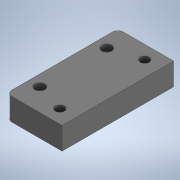
# Autodesk Inventor part: Stationaryjaw
Saved by Autodesk Inventor 2020.2 (Build 242310000, 310)
## iProperties
Created: 2021-06-22
Part Number: Stationaryjaw
Material: Generic
Document SubType Name: Modeling
Designer: JK
Density: 1 g/cm^3
Appearance: Gray
Author: JK
Autodesk Inventor part; units mm, degrees
ref_plane "YZ Plane" through (0, 0, 0) normal (1, 0, 0) x (0, 1, 0)
ref_plane "XZ Plane" through (0, 0, 0) normal (0, 1, 0) x (-1, 0, 0)
ref_plane "XY Plane" through (0, 0, 0) normal (0, 0, 1) x (1, 0, 0)
sketch "Sketch1" plane through (0, 0, 0) normal (0, 1, 0) x (-1, 0, 0)
  line L0 (25, 50) -> (-25, 50)
  line L1 (-25, 50) -> (-25, -50)
  line L2 (-25, -50) -> (25, -50)
  line L3 (25, -50) -> (25, 50)
  line L4 (25, 50) -> (-25, -50) construction
  line L5 (-25, 50) -> (25, -50) construction
  circle A0 centre (-11, 38) radius 6.5
  circle A1 centre (-11, -38) radius 6.5
  point P0 (0, 0)
  dimension "d0" = 13
  dimension "d1" = 100
  dimension "d2" = 50
  dimension "d3" = 14
  dimension "d4" = 12
  dimension "d5" = 12
  constraints: 12 end point, 2 centre point, 2 midpoint, 2 parallel, 1 equal radius, 1 horizontal, 1 perpendicular, 1 vertical alignment
  measures "d0" diameter of A0
  measures "d1" distance of L2.end L0.start
  measures "d2" distance of L1.end L2.end
  measures "d3" distance from line of A0.centre L1
  measures "d4" distance from line of L0 A0.centre
  measures "d5" distance from line of L2 A1.centre
extrude "Extrusion1" add sketch "Sketch1" along normal blind 20
sketch "Sketch2" plane through (0, 20, 0) normal (0, 1, 0) x (1, 0, 0)
  circle A0 centre (11, -38) radius 6.5 projected
  circle A1 centre (11, -38) radius 4
  circle A2 centre (11, 38) radius 6.5 projected
  circle A3 centre (11, 38) radius 4
  point P0 (0, 0)
  dimension "d8" = 8
  dimension "d9" = 8
  constraints: 2 centre point, 2 coincident
  measures "d8" diameter of A1
  measures "d9" diameter of A3
extrude "Extrusion2" add sketch "Sketch2" against normal blind 5
sketch "Sketch3" plane through (0, 0, 0) normal (0, -1, 0) x (1, 0, 0)
  circle A0 centre (-15, -30) radius 2.65
  circle A1 centre (-15, 30) radius 2.65
  line L0 (-25, -50) -> (-25, 50) projected
  line L1 (25, -50) -> (-25, -50) projected
  line L2 (-25, 50) -> (25, 50) projected
  point P0 (0, 0)
  dimension "d12" = 5.3
  dimension "d13" = 10
  dimension "d14" = 20
  dimension "d15" = 20
  dimension "d16" = 10
  constraints: 2 centre point, 1 equal radius
  measures "d12" diameter of A0
  measures "d13" distance from line of L0 A0.centre
  measures "d14" distance from line of L1 A0.centre
  measures "d15" distance from line of L2 A1.centre
  measures "d16" distance from line of L0 A1.centre
extrude "Extrusion3" cut sketch "Sketch3" against normal through all
fillet "Fillet1" radius 5 2 edges at (-25, 10, -50) (-25, 10, 50)
sketch "Sketch4" plane through (0, 20, 0) normal (0, 1, 0) x (1, 0, 0)
  circle A0 centre (-15, -30) radius 2.65 projected
  line L0 (-19.734, -29.95) -> (-17.3237, -25.8752)
  line L1 (-17.3237, -25.8752) -> (-12.5897, -25.9252)
  line L2 (-12.5897, -25.9252) -> (-10.266, -30.05)
  line L3 (-10.266, -30.05) -> (-12.6763, -34.1248)
  line L4 (-12.6763, -34.1248) -> (-17.4103, -34.0748)
  line L5 (-17.4103, -34.0748) -> (-19.734, -29.95)
  circle A1 centre (-15, -30) radius 4.1
  circle A2 centre (-15, 30) radius 2.65 projected
  line L6 (-19.7332, 30.1003) -> (-17.2797, 34.1492)
  line L7 (-17.2797, 34.1492) -> (-12.5465, 34.0489)
  line L8 (-12.5465, 34.0489) -> (-10.2668, 29.8997)
  line L9 (-10.2668, 29.8997) -> (-12.7203, 25.8508)
  line L10 (-12.7203, 25.8508) -> (-17.4535, 25.9511)
  line L11 (-17.4535, 25.9511) -> (-19.7332, 30.1003)
  circle A3 centre (-15, 30) radius 4.1
  point P0 (0, 0)
  dimension "d20" = 8.2
  constraints: 24 end point, 4 coincident, 2 centre point, 2 tangent, 1 equal radius, 26 other
  measures "d20" diameter of A1
extrude "Extrusion4" [suppressed]
sketch "Sketch5" plane through (25, 0, 50) normal (1, 0, 0) x (0, 0, -1)
  line L0 (100, 0) -> (100, 20) projected
  line L1 (100, 20) -> (120, 20)
  line L2 (120, 20) -> (120, 0)
  line L3 (120, 0) -> (100, 0)
  line L4 (100, 0) -> (100, 20)
  circle A0 centre (110, 10) radius 2.75
  line L5 (0, 0) -> (0, 20) projected
  line L6 (0, 0) -> (-20, 0)
  line L7 (-20, 0) -> (-20, 20)
  line L8 (-20, 20) -> (0, 20)
  line L9 (0, 20) -> (0, 0)
  circle A1 centre (-10, 10) radius 2.75
  point P0 (50, 0)
  point P1 (0, 20)
  dimension "d23" = 20
  dimension "d24" = 5.5
  dimension "d27" = 20
  dimension "d28" = 20
  dimension "d29" = 20
  dimension "d30" = 5.5
  constraints: 16 end point, 4 parallel, 2 centre point, 2 horizontal, 2 perpendicular
  measures "d23" distance between parallel lines of L2 L0
  measures "d24" diameter of A0
  measures "d27" distance between parallel lines of L7 L5
  measures "d28" distance between parallel lines of L6 L8
  measures "d29" distance between parallel lines of L3 L1
  measures "d30" diameter of A1
extrude "Extrusion5" [suppressed]
chamfer "Chamfer1" [suppressed]
sketch "Sketch6" plane through (5, 0, 50) normal (-1, 0, 0) x (0, 0, 1)
  arc A0 (-110, 12.75) -> (-110, 7.25) centre (-110, 10) ccw projected
  circle A1 centre (-110, 10) radius 4.75
  circle A2 centre (10, 10) radius 2.75 projected
  circle A3 centre (10, 10) radius 4.75
  point P0 (-50, 0)
  dimension "d34" = 9.5
  constraints: 2 centre point, 2 coincident, 1 equal radius
  measures "d34" diameter of A3
extrude "Extrusion6" [suppressed]
fillet "Fillet2" [suppressed]
sketch "Sketch7" plane through (0, 20, 0) normal (0, 1, 0) x (1, 0, 0)
  circle A0 centre (-15, 30) radius 2.65 projected
  circle A1 centre (-15, 30) radius 4.5
  circle A2 centre (-15, -30) radius 2.65 projected
  circle A3 centre (-15, -30) radius 4.5
  point P0 (0, 0)
  dimension "d38" = 9
  constraints: 2 centre point, 2 coincident, 1 equal radius
  measures "d38" diameter of A1
extrude "Extrusion7" cut sketch "Sketch7" against normal blind 5 contours A0 | A1 | A2 | A3
sketch "Sketch8" plane through (0, 0, 0) normal (0, -1, 0) x (1, 0, 0)
  circle A0 centre (11, 0) radius 4.1
  circle A1 centre (11, -38) radius 6.5 projected
  line L0 (25, 50) -> (25, -50) projected
  line L1 (-20, 50) -> (25, 50) projected
  arc A2 (-20, 50) -> (-25, 45) centre (-20, 45) ccw projected
  line L2 (-25, -45) -> (-25, 45) projected
  arc A3 (-25, -45) -> (-20, -50) centre (-20, -45) ccw projected
  line L3 (25, -50) -> (-20, -50) projected
  circle A4 centre (-15, 30) radius 2.65 projected
  circle A5 centre (-15, -30) radius 2.65 projected
  circle A6 centre (11, 38) radius 6.5 projected
  circle A7 centre (11, -38) radius 6.5 projected
  point P0 (0, 0)
  dimension "d41" = 8.2
  constraints: 1 centre point, 1 vertical alignment
  measures "d41" diameter of A0
extrude "Extrusion8" cut sketch "Sketch8" against normal blind 10 contours A0
body "Solid1"
